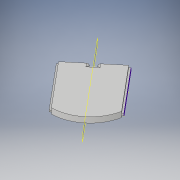
# Autodesk Inventor part: buzzerLid3
Saved by Autodesk Inventor 2019 (Build 230136000, 136)
## iProperties
Created: 2019-06-15
Part Number: buzzerLid3
Material: Generic
Document SubType Name: Modeling
Designer: Owner
Density: 1 g/cm^3
Appearance: Default
Author: Owner
Autodesk Inventor part; units mm, degrees
ref_plane "YZ Plane" through (0, 0, 0) normal (1, 0, 0) x (0, 1, 0)
ref_plane "XZ Plane" through (0, 0, 0) normal (0, 1, 0) x (-1, 0, 0)
ref_plane "XY Plane" through (0, 0, 0) normal (0, 0, 1) x (1, 0, 0)
sketch "Sketch1" plane through (0, 0, 0) normal (0, 1, 0) x (-1, 0, 0)
  circle A0 centre (0, 0) radius 50
  arc A1 (-0.8192, 49.9933) -> (-49.0545, 9.6775) centre (0, 0) ccw
  line L0 (-0.8192, 49.9933) -> (-49.0545, 9.6775)
  line L1 (-49.0545, 9.6775) -> (-3.176, -45.2133)
  line L2 (-3.176, -45.2133) -> (45.0593, -4.8975)
  line L3 (45.0593, -4.8975) -> (-0.8192, 49.9933)
  dimension "d0" = 100
  dimension "d1" = 62.865
  dimension "d2" = 71.5391
  constraints: 8 end point, 4 point on circle, 2 centre point, 2 parallel, 1 coincident, 1 concentric, 1 perpendicular
  measures "d0" diameter of A0
  measures "d1" distance of L0.start L0.end
  measures "d2" distance of L1.end L0.end
extrude "Extrusion1" add sketch "Sketch1" along normal blind 6.858 contours L0 A0 | L3 L2 L1 L0
sketch "Sketch2" plane through (3.176, 0, -45.2133) normal (0.7672841, 0, -0.6413074) x (-0.6413074, 0, -0.7672841)
  line L0 (-71.5391, 0) -> (-82.6547, 0) projected
  line L1 (-71.5391, 0) -> (-71.5391, 2.159)
  line L2 (-71.5391, 0) -> (-71.5391, 6.858) projected
  line L3 (-71.5391, 2.159) -> (-71.5391, 4.318)
  line L4 (-71.5391, 2.159) -> (-71.5391, 4.318)
  line L5 (-71.5391, 4.318) -> (0.0381, 4.318)
  line L6 (0.0381, 4.318) -> (0.0381, 2.159)
  line L7 (0.0381, 2.159) -> (-71.5391, 2.159)
  point P0 (-32.6547, 0)
  dimension "d5" = 2.159
  dimension "d6" = 2.159
  constraints: 12 end point, 2 parallel, 2 point on line, 1 collinear, 1 perpendicular
  measures "d5" distance of L0.start L1.end
  measures "d6" distance of L1.end L3.end
extrude "Extrusion2" add sketch "Sketch2" along normal blind 2.032
ref_plane "Work Plane1" through (-20.9417, 6.858, -25.0554) normal (-0.7672841, 0, 0.6413074) x (0.6413074, 0, 0.7672841)
mirror "Mirror1" about plane through (-20.9417, 6.858, -25.0554) normal (-0.7672841, 0, 0.6413074) of "Extrusion2"
sketch "Sketch3" plane through (0, 6.858, 0) normal (0, 1, 0) x (1, 0, 0)
  line L0 (3.176, 45.2133) -> (-45.0593, 4.8975) projected
  line L1 (-20.9417, 25.0554) -> (-23.865, 22.612)
  line L2 (-23.865, 22.612) -> (-21.4217, 19.6887)
  line L3 (-21.4217, 19.6887) -> (-18.4983, 22.1321)
  line L4 (-18.4983, 22.1321) -> (-20.9417, 25.0554)
  line L5 (-20.9417, 25.0554) -> (-18.0183, 27.4988)
  line L6 (-18.0183, 27.4988) -> (-15.575, 24.5754)
  line L7 (-15.575, 24.5754) -> (-18.4983, 22.1321)
  line L8 (-18.4983, 22.1321) -> (-20.9417, 25.0554)
  point P0 (0, 0)
  dimension "d9" = 3.81
  dimension "d10" = 3.81
  dimension "d11" = 3.81
  constraints: 16 end point, 4 parallel, 2 perpendicular, 2 point on line, 1 midpoint
  measures "d9" distance of L1.start L1.end
  measures "d10" distance of L2.end L1.end
  measures "d11" distance of L1.start L5.end
extrude "Extrusion3" cut sketch "Sketch3" against normal blind 2.54
chamfer "Chamfer1" distance 2.54 angle 45 1 edges at (-20.9417, 4.318, -25.0554)
fillet "Fillet1" radius 3.175 1 edges at (-18.4983, 4.318, -22.1321)
fillet "Fillet2" radius 3.175 1 edges at (-19.3128, 4.318, -23.1065)
fillet "Fillet3" radius 2.54 1 edges at (-18.4983, 6.858, -22.1321)
fillet "Fillet4" radius 2.54 2 edges at (-20.7981, 6.858, -18.9427) (-22.6434, 6.858, -21.1504)
fillet "Fillet5" radius 2.54 2 edges at (-14.9514, 6.858, -23.8294) (-16.7966, 6.858, -26.0371)
fillet "Fillet6" radius 2.54 1 edges at (-20.9417, 1.778, -25.0554)
sketch "Sketch4" plane through (0, 0, 0) normal (0, -1, 0) x (1, 0, 0)
  point P0 (0, 0)
sketch "Sketch5" plane through (4.7351, 0, -46.5164) normal (0.7672841, 0, -0.6413074) x (-0.6413074, 0, -0.7672841)
  line L0 (-71.5391, 2.159) -> (-71.5391, 4.318) projected
  line L1 (-71.5391, 2.159) -> (0, 2.159) projected
  line L2 (-71.5391, 4.318) -> (0, 4.318)
  line L3 (0, 4.318) -> (0, 2.159)
  line L4 (0, 2.159) -> (-71.5391, 2.159)
  line L5 (-71.5391, 2.159) -> (-71.5391, 4.318)
  point P0 (-32.6547, 0)
  constraints: 8 end point, 2 parallel, 1 horizontal, 1 perpendicular
body "Solid1"
